Autodesk Fusion 360 part; units mm, degrees
(part 6 of 9)
  spline S17 degree 5 poles (27.8077, 5.2259) (27.7982, 5.2278) (27.7791, 5.232) (27.7507, 5.2389) (27.7131, 5.2496) (27.6667, 5.2648) (27.6206, 5.2814) (27.5747, 5.2988) (27.529, 5.3167) (27.4833, 5.3349) (27.4376, 5.3534) (27.3921, 5.3724) (27.3468, 5.3919) (27.3016, 5.4121) (27.2567, 5.4329) (27.2119, 5.4544) (27.1672, 5.4764) (27.1227, 5.4988) (27.0784, 5.5216) (27.0341, 5.5447) (26.9899, 5.5683) (26.9459, 5.5922) (26.902, 5.6164) (26.8582, 5.6411) (26.8146, 5.6662) (26.771, 5.6917) (26.7277, 5.7176) (26.6844, 5.7438) (26.6412, 5.7703) (26.5982, 5.7972) (26.5553, 5.8244) (26.5125, 5.8519) (26.4698, 5.8797) (26.4272, 5.9079) (26.3848, 5.9363) (26.3425, 5.9651) (26.3003, 5.9942) (26.2582, 6.0236) (26.2162, 6.0533) (26.1743, 6.0833) (26.1326, 6.1136) (26.091, 6.1441) (26.0495, 6.1749) (26.0081, 6.2061) (25.9668, 6.2375) (25.9256, 6.2691) (25.8846, 6.3011) (25.8437, 6.3333) (25.8029, 6.3658) (25.7622, 6.3985) (25.7216, 6.4315) (25.6811, 6.4648) (25.6408, 6.4983) (25.6005, 6.5321) (25.5604, 6.5661) (25.5204, 6.6004) (25.4805, 6.6349) (25.4408, 6.6696) (25.4011, 6.7047) (25.3616, 6.7399) (25.3222, 6.7754) (25.2829, 6.8111) (25.2437, 6.8471) (25.2046, 6.8833) (25.1657, 6.9197) (25.1269, 6.9564) (25.0882, 6.9933) (25.0496, 7.0304) (25.0111, 7.0677) (24.9727, 7.1053) (24.9345, 7.1431) (24.904, 7.1735) (24.8812, 7.1964) (24.866, 7.2117) (24.8584, 7.2194) knots 0 0 0 0 0 0 0.01428571 0.02857143 0.04285714 0.05714286 0.07142857 0.08571429 0.1 0.11428571 0.12857143 0.14285714 0.15714286 0.17142857 0.18571429 0.2 0.21428571 0.22857143 0.24285714 0.25714286 0.27142857 0.28571429 0.3 0.31428571 0.32857143 0.34285714 0.35714286 0.37142857 0.38571429 0.4 0.41428571 0.42857143 0.44285714 0.45714286 0.47142857 0.48571429 0.5 0.51428571 0.52857143 0.54285714 0.55714286 0.57142857 0.58571429 0.6 0.61428571 0.62857143 0.64285714 0.65714286 0.67142857 0.68571429 0.7 0.71428571 0.72857143 0.74285714 0.75714286 0.77142857 0.78571429 0.8 0.81428571 0.82857143 0.84285714 0.85714286 0.87142857 0.88571429 0.9 0.91428571 0.92857143 0.94285714 0.95714286 0.97142857 0.98571429 1 1 1 1 1 1
  line L17 (27.8077, 5.2259) -> (27.9539, 5.196)
  arc A35 (28.7419, 4.0645) -> (27.9539, 5.196) centre (27.7535, 4.2163) ccw
  arc A36 (28.7419, 4.0645) -> (28.689, 3.6964) centre (48.0648, 1.0985) ccw
  arc A37 (27.6141, 2.8328) -> (28.689, 3.6964) centre (27.6978, 3.8293) ccw
  line L18 (27.6141, 2.8328) -> (27.4655, 2.8453)
  spline S18 degree 5 poles (27.4655, 2.8453) (27.4557, 2.8461) (27.4363, 2.8475) (27.407, 2.8489) (27.368, 2.8492) (27.3192, 2.8477) (27.2703, 2.8448) (27.2214, 2.841) (27.1724, 2.8367) (27.1234, 2.8321) (27.0744, 2.8272) (27.0254, 2.8218) (26.9764, 2.8159) (26.9274, 2.8092) (26.8784, 2.8019) (26.8294, 2.7939) (26.7803, 2.7854) (26.7313, 2.7764) (26.6823, 2.7671) (26.6333, 2.7573) (26.5843, 2.7472) (26.5353, 2.7367) (26.4864, 2.7257) (26.4374, 2.7144) (26.3885, 2.7026) (26.3395, 2.6904) (26.2906, 2.6778) (26.2417, 2.6649) (26.1928, 2.6516) (26.144, 2.6379) (26.0951, 2.6239) (26.0463, 2.6096) (25.9975, 2.5949) (25.9487, 2.5799) (25.9, 2.5645) (25.8513, 2.5488) (25.8026, 2.5328) (25.7539, 2.5165) (25.7053, 2.4998) (25.6567, 2.4828) (25.6081, 2.4655) (25.5595, 2.4479) (25.511, 2.43) (25.4625, 2.4118) (25.4141, 2.3933) (25.3657, 2.3746) (25.3173, 2.3555) (25.269, 2.3361) (25.2206, 2.3164) (25.1724, 2.2965) (25.1241, 2.2762) (25.0759, 2.2557) (25.0278, 2.2349) (24.9797, 2.2139) (24.9316, 2.1925) (24.8836, 2.1709) (24.8356, 2.149) (24.7876, 2.1269) (24.7397, 2.1045) (24.6919, 2.0818) (24.644, 2.0588) (24.5963, 2.0356) (24.5485, 2.0122) (24.5009, 1.9884) (24.4532, 1.9644) (24.4057, 1.9402) (24.3581, 1.9157) (24.3106, 1.891) (24.2632, 1.866) (24.2158, 1.8408) (24.1685, 1.8153) (24.1307, 1.7947) (24.1023, 1.7791) (24.0834, 1.7687) (24.074, 1.7635) knots 0 0 0 0 0 0 0.01428571 0.02857143 0.04285714 0.05714286 0.07142857 0.08571429 0.1 0.11428571 0.12857143 0.14285714 0.15714286 0.17142857 0.18571429 0.2 0.21428571 0.22857143 0.24285714 0.25714286 0.27142857 0.28571429 0.3 0.31428571 0.32857143 0.34285714 0.35714286 0.37142857 0.38571429 0.4 0.41428571 0.42857143 0.44285714 0.45714286 0.47142857 0.48571429 0.5 0.51428571 0.52857143 0.54285714 0.55714286 0.57142857 0.58571429 0.6 0.61428571 0.62857143 0.64285714 0.65714286 0.67142857 0.68571429 0.7 0.71428571 0.72857143 0.74285714 0.75714286 0.77142857 0.78571429 0.8 0.81428571 0.82857143 0.84285714 0.85714286 0.87142857 0.88571429 0.9 0.91428571 0.92857143 0.94285714 0.95714286 0.97142857 0.98571429 1 1 1 1 1 1
  arc A38 (24.074, 1.7635) -> (24.074, 0.4334) centre (48.0648, 1.0985) ccw
  spline S19 degree 5 poles (27.4655, -0.6484) (27.4557, -0.6492) (27.4363, -0.6506) (27.407, -0.6519) (27.368, -0.6523) (27.3192, -0.6508) (27.2703, -0.6479) (27.2214, -0.6441) (27.1724, -0.6398) (27.1234, -0.6352) (27.0744, -0.6303) (27.0254, -0.6249) (26.9764, -0.6189) (26.9274, -0.6123) (26.8784, -0.605) (26.8294, -0.597) (26.7803, -0.5885) (26.7313, -0.5795) (26.6823, -0.5701) (26.6333, -0.5604) (26.5843, -0.5503) (26.5353, -0.5398) (26.4864, -0.5288) (26.4374, -0.5175) (26.3885, -0.5057) (26.3395, -0.4935) (26.2906, -0.4809) (26.2417, -0.468) (26.1928, -0.4546) (26.144, -0.441) (26.0951, -0.427) (26.0463, -0.4127) (25.9975, -0.398) (25.9487, -0.383) (25.9, -0.3676) (25.8513, -0.3519) (25.8026, -0.3359) (25.7539, -0.3195) (25.7053, -0.3029) (25.6567, -0.2859) (25.6081, -0.2686) (25.5595, -0.251) (25.511, -0.2331) (25.4625, -0.2149) (25.4141, -0.1964) (25.3657, -0.1776) (25.3173, -0.1585) (25.269, -0.1392) (25.2206, -0.1195) (25.1724, -0.0995) (25.1241, -0.0793) (25.0759, -0.0588) (25.0278, -0.038) (24.9797, -0.0169) (24.9316, 0.0044) (24.8836, 0.026) (24.8356, 0.0479) (24.7876, 0.0701) (24.7397, 0.0925) (24.6919, 0.1152) (24.644, 0.1381) (24.5963, 0.1613) (24.5485, 0.1848) (24.5009, 0.2085) (24.4532, 0.2325) (24.4057, 0.2567) (24.3581, 0.2812) (24.3106, 0.306) (24.2632, 0.3309) (24.2158, 0.3562) (24.1685, 0.3817) (24.1307, 0.4023) (24.1023, 0.4178) (24.0834, 0.4282) (24.074, 0.4334) knots 0 0 0 0 0 0 0.01428571 0.02857143 0.04285714 0.05714286 0.07142857 0.08571429 0.1 0.11428571 0.12857143 0.14285714 0.15714286 0.17142857 0.18571429 0.2 0.21428571 0.22857143 0.24285714 0.25714286 0.27142857 0.28571429 0.3 0.31428571 0.32857143 0.34285714 0.35714286 0.37142857 0.38571429 0.4 0.41428571 0.42857143 0.44285714 0.45714286 0.47142857 0.48571429 0.5 0.51428571 0.52857143 0.54285714 0.55714286 0.57142857 0.58571429 0.6 0.61428571 0.62857143 0.64285714 0.65714286 0.67142857 0.68571429 0.7 0.71428571 0.72857143 0.74285714 0.75714286 0.77142857 0.78571429 0.8 0.81428571 0.82857143 0.84285714 0.85714286 0.87142857 0.88571429 0.9 0.91428571 0.92857143 0.94285714 0.95714286 0.97142857 0.98571429 1 1 1 1 1 1
  line L19 (27.4655, -0.6484) -> (27.6141, -0.6359)
  arc A39 (28.689, -1.4995) -> (27.6141, -0.6359) centre (27.6978, -1.6324) ccw
  arc A40 (28.689, -1.4995) -> (28.7419, -1.8676) centre (48.0648, 1.0985) ccw
  arc A41 (27.9539, -2.999) -> (28.7419, -1.8676) centre (27.7535, -2.0193) ccw
  line L20 (27.9539, -2.999) -> (27.8077, -3.0289)
  spline S20 degree 5 poles (27.8077, -3.0289) (27.7982, -3.0309) (27.7791, -3.035) (27.7507, -3.042) (27.7131, -3.0526) (27.6667, -3.0678) (27.6206, -3.0844) (27.5747, -3.1018) (27.529, -3.1197) (27.4833, -3.138) (27.4376, -3.1565) (27.3921, -3.1755) (27.3468, -3.195) (27.3016, -3.2152) (27.2567, -3.236) (27.2119, -3.2575) (27.1672, -3.2794) (27.1227, -3.3019) (27.0784, -3.3247) (27.0341, -3.3478) (26.9899, -3.3713) (26.9459, -3.3952) (26.902, -3.4195) (26.8582, -3.4442) (26.8146, -3.4693) (26.771, -3.4948) (26.7277, -3.5206) (26.6844, -3.5468) (26.6412, -3.5734) (26.5982, -3.6002) (26.5553, -3.6274) (26.5125, -3.6549) (26.4698, -3.6828) (26.4272, -3.7109) (26.3848, -3.7394) (26.3425, -3.7682) (26.3003, -3.7973) (26.2582, -3.8267) (26.2162, -3.8564) (26.1743, -3.8864) (26.1326, -3.9166) (26.091, -3.9472) (26.0495, -3.978) (26.0081, -4.0091) (25.9668, -4.0405) (25.9256, -4.0722) (25.8846, -4.1042) (25.8437, -4.1364) (25.8029, -4.1688) (25.7622, -4.2016) (25.7216, -4.2346) (25.6811, -4.2678) (25.6408, -4.3014) (25.6005, -4.3351) (25.5604, -4.3692) (25.5204, -4.4034) (25.4805, -4.438) (25.4408, -4.4727) (25.4011, -4.5077) (25.3616, -4.543) (25.3222, -4.5785) (25.2829, -4.6142) (25.2437, -4.6501) (25.2046, -4.6863) (25.1657, -4.7228) (25.1269, -4.7594) (25.0882, -4.7963) (25.0496, -4.8334) (25.0111, -4.8708) (24.9727, -4.9083) (24.9345, -4.9461) (24.904, -4.9765) (24.8812, -4.9994) (24.866, -5.0148) (24.8584, -5.0224) knots 0 0 0 0 0 0 0.01428571 0.02857143 0.04285714 0.05714286 0.07142857 0.08571429 0.1 0.11428571 0.12857143 0.14285714 0.15714286 0.17142857 0.18571429 0.2 0.21428571 0.22857143 0.24285714 0.25714286 0.27142857 0.28571429 0.3 0.31428571 0.32857143 0.34285714 0.35714286 0.37142857 0.38571429 0.4 0.41428571 0.42857143 0.44285714 0.45714286 0.47142857 0.48571429 0.5 0.51428571 0.52857143 0.54285714 0.55714286 0.57142857 0.58571429 0.6 0.61428571 0.62857143 0.64285714 0.65714286 0.67142857 0.68571429 0.7 0.71428571 0.72857143 0.74285714 0.75714286 0.77142857 0.78571429 0.8 0.81428571 0.82857143 0.84285714 0.85714286 0.87142857 0.88571429 0.9 0.91428571 0.92857143 0.94285714 0.95714286 0.97142857 0.98571429 1 1 1 1 1 1
  arc A42 (24.8584, -5.0224) -> (25.2332, -6.2986) centre (48.0648, 1.0985) ccw
  spline S21 degree 5 poles (28.792, -6.3811) (28.7829, -6.3847) (28.7646, -6.3915) (28.737, -6.401) (28.6996, -6.4123) (28.6523, -6.4246) (28.6046, -6.4356) (28.5566, -6.4458) (28.5084, -6.4555) (28.4601, -6.4648) (28.4117, -6.4739) (28.3632, -6.4825) (28.3145, -6.4906) (28.2656, -6.4981) (28.2165, -6.5048) (28.1672, -6.511) (28.1178, -6.5167) (28.0682, -6.5219) (28.0186, -6.5267) (27.9688, -6.5311) (27.9189, -6.5352) (27.869, -6.5389) (27.8189, -6.5422) (27.7687, -6.5451) (27.7184, -6.5476) (27.6681, -6.5497) (27.6176, -6.5514) (27.567, -6.5528) (27.5164, -6.5538) (27.4656, -6.5544) (27.4148, -6.5548) (27.364, -6.5548) (27.313, -6.5544) (27.262, -6.5538) (27.2109, -6.5527) (27.1597, -6.5514) (27.1085, -6.5498) (27.0572, -6.5478) (27.0058, -6.5455) (26.9544, -6.5429) (26.9029, -6.54) (26.8514, -6.5368) (26.7998, -6.5333) (26.7481, -6.5295) (26.6964, -6.5254) (26.6447, -6.521) (26.5929, -6.5163) (26.541, -6.5114) (26.4891, -6.5061) (26.4372, -6.5006) (26.3852, -6.4947) (26.3332, -6.4886) (26.2811, -6.4822) (26.229, -6.4756) (26.1769, -6.4687) (26.1247, -6.4614) (26.0725, -6.454) (26.0202, -6.4462) (25.968, -6.4382) (25.9157, -6.4299) (25.8633, -6.4214) (25.8109, -6.4126) (25.7585, -6.4035) (25.7061, -6.3942) (25.6536, -6.3846) (25.6012, -6.3747) (25.5487, -6.3646) (25.4961, -6.3543) (25.4436, -6.3436) (25.391, -6.3328) (25.3384, -6.3217) (25.2963, -6.3126) (25.2647, -6.3056) (25.2437, -6.301) (25.2332, -6.2986) knots 0 0 0 0 0 0 0.01428571 0.02857143 0.04285714 0.05714286 0.07142857 0.08571429 0.1 0.11428571 0.12857143 0.14285714 0.15714286 0.17142857 0.18571429 0.2 0.21428571 0.22857143 0.24285714 0.25714286 0.27142857 0.28571429 0.3 0.31428571 0.32857143 0.34285714 0.35714286 0.37142857 0.38571429 0.4 0.41428571 0.42857143 0.44285714 0.45714286 0.47142857 0.48571429 0.5 0.51428571 0.52857143 0.54285714 0.55714286 0.57142857 0.58571429 0.6 0.61428571 0.62857143 0.64285714 0.65714286 0.67142857 0.68571429 0.7 0.71428571 0.72857143 0.74285714 0.75714286 0.77142857 0.78571429 0.8 0.81428571 0.82857143 0.84285714 0.85714286 0.87142857 0.88571429 0.9 0.91428571 0.92857143 0.94285714 0.95714286 0.97142857 0.98571429 1 1 1 1 1 1
  line L21 (28.792, -6.3811) -> (28.9311, -6.3273)
  arc A43 (30.2058, -6.8531) -> (28.9311, -6.3273) centre (29.2922, -7.2598) ccw
  arc A44 (30.2058, -6.8531) -> (30.3603, -7.1913) centre (48.0648, 1.0985) ccw
  arc A45 (29.9229, -8.499) -> (30.3603, -7.1913) centre (29.4546, -7.6154) ccw
  line L22 (29.9229, -8.499) -> (29.7911, -8.5688)
  spline S22 degree 5 poles (29.7911, -8.5688) (29.7825, -8.5734) (29.7654, -8.5827) (29.74, -8.5974) (29.707, -8.6182) (29.6668, -8.6459) (29.6272, -8.6748) (29.5881, -8.7044) (29.5492, -8.7345) (29.5105, -8.7648) (29.472, -8.7955) (29.4336, -8.8265) (29.3956, -8.858) (29.358, -8.8901) (29.3207, -8.9228) (29.2838, -8.956) (29.2471, -8.9896) (29.2108, -9.0237) (29.1746, -9.0581) (29.1386, -9.0927) (29.1029, -9.1277) (29.0674, -9.1631) (29.0321, -9.1987) (28.997, -9.2348) (28.9622, -9.2712) (28.9277, -9.3079) (28.8933, -9.3449) (28.8592, -9.3822) (28.8252, -9.4198) (28.7915, -9.4577) (28.758, -9.4959) (28.7247, -9.5344) (28.6916, -9.5731) (28.6587, -9.6121) (28.626, -9.6514) (28.5935, -9.6909) (28.5612, -9.7307) (28.5291, -9.7708) (28.4972, -9.8111) (28.4654, -9.8517) (28.4339, -9.8925) (28.4026, -9.9335) (28.3715, -9.9748) (28.3405, -10.0163) (28.3097, -10.0581) (28.2792, -10.1001) (28.2488, -10.1423) (28.2186, -10.1847) (28.1886, -10.2274) (28.1588, -10.2703) (28.1291, -10.3134) (28.0997, -10.3567) (28.0704, -10.4002) (28.0413, -10.4439) (28.0124, -10.4879) (27.9837, -10.532) (27.9551, -10.5764) (27.9268, -10.621) (27.8986, -10.6657) (27.8706, -10.7107) (27.8428, -10.7558) (27.8151, -10.8012) (27.7877, -10.8467) (27.7604, -10.8925) (27.7333, -10.9384) (27.7064, -10.9845) (27.6796, -11.0308) (27.6531, -11.0773) (27.6267, -11.124) (27.6004, -11.1708) (27.5744, -11.2178) (27.5537, -11.2556) (27.5383, -11.284) (27.528, -11.303) (27.5229, -11.3125) knots 0 0 0 0 0 0 0.01428571 0.02857143 0.04285714 0.05714286 0.07142857 0.08571429 0.1 0.11428571 0.12857143 0.14285714 0.15714286 0.17142857 0.18571429 0.2 0.21428571 0.22857143 0.24285714 0.25714286 0.27142857 0.28571429 0.3 0.31428571 0.32857143 0.34285714 0.35714286 0.37142857 0.38571429 0.4 0.41428571 0.42857143 0.44285714 0.45714286 0.47142857 0.48571429 0.5 0.51428571 0.52857143 0.54285714 0.55714286 0.57142857 0.58571429 0.6 0.61428571 0.62857143 0.64285714 0.65714286 0.67142857 0.68571429 0.7 0.71428571 0.72857143 0.74285714 0.75714286 0.77142857 0.78571429 0.8 0.81428571 0.82857143 0.84285714 0.85714286 0.87142857 0.88571429 0.9 0.91428571 0.92857143 0.94285714 0.95714286 0.97142857 0.98571429 1 1 1 1 1 1
  arc A46 (27.5229, -11.3125) -> (28.242, -12.4314) centre (48.0648, 1.0985) ccw
  spline S23 degree 5 poles (31.68, -11.5079) (31.6722, -11.5139) (31.6566, -11.5256) (31.6327, -11.5425) (31.6001, -11.5639) (31.5582, -11.589) (31.5155, -11.613) (31.4723, -11.6363) (31.4288, -11.6591) (31.3851, -11.6817) (31.3412, -11.7041) (31.2971, -11.726) (31.2526, -11.7475) (31.2078, -11.7684) (31.1626, -11.7888) (31.117, -11.8086) (31.0712, -11.8279) (31.0251, -11.8469) (30.9788, -11.8655) (30.9323, -11.8838) (30.8856, -11.9017) (30.8387, -11.9194) (30.7916, -11.9367) (30.7443, -11.9536) (30.6968, -11.9701) (30.649, -11.9863) (30.601, -12.0022) (30.5529, -12.0177) (30.5046, -12.033) (30.4561, -12.0479) (30.4075, -12.0625) (30.3586, -12.0769) (30.3097, -12.0909) (30.2605, -12.1046) (30.2112, -12.118) (30.1617, -12.1312) (30.1121, -12.144) (30.0623, -12.1566) (30.0124, -12.1689) (29.9623, -12.1809) (29.9121, -12.1926) (29.8618, -12.204) (29.8113, -12.2152) (29.7606, -12.2261) (29.7099, -12.2367) (29.659, -12.2471) (29.608, -12.2572) (29.5568, -12.267) (29.5056, -12.2766) (29.4542, -12.2859) (29.4026, -12.295) (29.351, -12.3038) (29.2993, -12.3123) (29.2474, -12.3206) (29.1954, -12.3287) (29.1433, -12.3364) (29.0911, -12.344) (29.0388, -12.3513) (28.9864, -12.3583) (28.9338, -12.3651) (28.8812, -12.3717) (28.8285, -12.378) (28.7756, -12.384) (28.7227, -12.3898) (28.6697, -12.3954) (28.6165, -12.4007) (28.5633, -12.4058) (28.51, -12.4107) (28.4566, -12.4153) (28.4031, -12.4197) (28.3495, -12.4239) (28.3065, -12.427) (28.2743, -12.4292) (28.2528, -12.4307) (28.242, -12.4314) knots 0 0 0 0 0 0 0.01428571 0.02857143 0.04285714 0.05714286 0.07142857 0.08571429 0.1 0.11428571 0.12857143 0.14285714 0.15714286 0.17142857 0.18571429 0.2 0.21428571 0.22857143 0.24285714 0.25714286 0.27142857 0.28571429 0.3 0.31428571 0.32857143 0.34285714 0.35714286 0.37142857 0.38571429 0.4 0.41428571 0.42857143 0.44285714 0.45714286 0.47142857 0.48571429 0.5 0.51428571 0.52857143 0.54285714 0.55714286 0.57142857 0.58571429 0.6 0.61428571 0.62857143 0.64285714 0.65714286 0.67142857 0.68571429 0.7 0.71428571 0.72857143 0.74285714 0.75714286 0.77142857 0.78571429 0.8 0.81428571 0.82857143 0.84285714 0.85714286 0.87142857 0.88571429 0.9 0.91428571 0.92857143 0.94285714 0.95714286 0.97142857 0.98571429 1 1 1 1 1 1
  line L23 (31.68, -11.5079) -> (31.7982, -11.4171)
  arc A47 (33.1694, -11.5624) -> (31.7982, -11.4171) centre (32.4074, -12.2101) ccw
  arc A48 (33.1694, -11.5624) -> (33.4129, -11.8435) centre (48.0648, 1.0985) ccw
  arc A49 (33.3617, -13.2214) -> (33.4129, -11.8435) centre (32.6634, -12.5055) ccw
  line L24 (33.3617, -13.2214) -> (33.2549, -13.3255)
  spline S24 degree 5 poles (33.2549, -13.3255) (33.2479, -13.3323) (33.2341, -13.3461) (33.214, -13.3673) (33.1881, -13.3966) (33.1573, -13.4345) (33.1275, -13.4734) (33.0983, -13.5128) (33.0695, -13.5526) (33.0409, -13.5926) (33.0125, -13.6329) (32.9845, -13.6735) (32.9569, -13.7144) (32.9298, -13.7558) (32.9033, -13.7976) (32.8772, -13.8399) (32.8515, -13.8825) (32.8262, -13.9254) (32.8012, -13.9686) (32.7765, -14.012) (32.752, -14.0557) (32.7279, -14.0996) (32.7041, -14.1438) (32.6806, -14.1882) (32.6575, -14.2329) (32.6346, -14.2779) (32.6121, -14.3231) (32.5899, -14.3685) (32.5679, -14.4142) (32.5463, -14.46) (32.5248, -14.5061) (32.5037, -14.5524) (32.4829, -14.5989) (32.4623, -14.6456) (32.442, -14.6925) (32.4219, -14.7396) (32.4021, -14.7869) (32.3826, -14.8344) (32.3634, -14.882) (32.3444, -14.9299) (32.3256, -14.9779) (32.3071, -15.0261) (32.2889, -15.0745) (32.2709, -15.1231) (32.2531, -15.1718) (32.2356, -15.2207) (32.2184, -15.2698) (32.2014, -15.319) (32.1846, -15.3684) (32.168, -15.4179) (32.1518, -15.4676) (32.1357, -15.5175) (32.1199, -15.5675) (32.1043, -15.6177) (32.0889, -15.668) (32.0738, -15.7184) (32.0589, -15.769) (32.0443, -15.8198) (32.0298, -15.8707) (32.0156, -15.9217) (32.0017, -15.9728) (31.9879, -16.0241) (31.9744, -16.0756) (31.9611, -16.1272) (31.948, -16.1789) (31.9352, -16.2307) (31.9226, -16.2826) (31.9102, -16.3347) (31.898, -16.3869) (31.8861, -16.4393) (31.8743, -16.4917) (31.8651, -16.5338) (31.8583, -16.5654) (31.8538, -16.5865) (31.8516, -16.5971) knots 0 0 0 0 0 0 0.01428571 0.02857143 0.04285714 0.05714286 0.07142857 0.08571429 0.1 0.11428571 0.12857143 0.14285714 0.15714286 0.17142857 0.18571429 0.2 0.21428571 0.22857143 0.24285714 0.25714286 0.27142857 0.28571429 0.3 0.31428571 0.32857143 0.34285714 0.35714286 0.37142857 0.38571429 0.4 0.41428571 0.42857143 0.44285714 0.45714286 0.47142857 0.48571429 0.5 0.51428571 0.52857143 0.54285714 0.55714286 0.57142857 0.58571429 0.6 0.61428571 0.62857143 0.64285714 0.65714286 0.67142857 0.68571429 0.7 0.71428571 0.72857143 0.74285714 0.75714286 0.77142857 0.78571429 0.8 0.81428571 0.82857143 0.84285714 0.85714286 0.87142857 0.88571429 0.9 0.91428571 0.92857143 0.94285714 0.95714286 0.97142857 0.98571429 1 1 1 1 1 1
  arc A50 (31.8516, -16.5971) -> (32.8568, -17.4681) centre (48.0648, 1.0985) ccw
  spline S25 degree 5 poles (35.8953, -15.6134) (35.8895, -15.6213) (35.8778, -15.6369) (35.8597, -15.6599) (35.8344, -15.6896) (35.8013, -15.7255) (35.7671, -15.7606) (35.7322, -15.7951) (35.6969, -15.8293) (35.6613, -15.8633) (35.6255, -15.8971) (35.5894, -15.9306) (35.5528, -15.9637) (35.5156, -15.9964) (35.478, -16.0286) (35.4399, -16.0605) (35.4013, -16.0919) (35.3625, -16.1231) (35.3233, -16.154) (35.2838, -16.1847) (35.2441, -16.2151) (35.2041, -16.2452) (35.1637, -16.2751) (35.1231, -16.3046) (35.0821, -16.3339) (35.0409, -16.3629) (34.9993, -16.3916) (34.9575, -16.4201) (34.9155, -16.4483) (34.8732, -16.4763) (34.8306, -16.5041) (34.7878, -16.5316) (34.7447, -16.5588) (34.7014, -16.5858) (34.6579, -16.6126) (34.6141, -16.6392) (34.5701, -16.6655) (34.5259, -16.6915) (34.4815, -16.7174) (34.4368, -16.743) (34.3919, -16.7684) (34.3469, -16.7936) (34.3016, -16.8185) (34.2561, -16.8432) (34.2103, -16.8677) (34.1644, -16.892) (34.1183, -16.9161) (34.072, -16.9399) (34.0255, -16.9636) (33.9788, -16.987) (33.932, -17.0102) (33.8849, -17.0332) (33.8376, -17.056) (33.7902, -17.0785) (33.7426, -17.1009) (33.6948, -17.123) (33.6468, -17.145) (33.5987, -17.1667) (33.5504, -17.1882) (33.5019, -17.2095) (33.4532, -17.2307) (33.4044, -17.2516) (33.3554, -17.2723) (33.3063, -17.2928) (33.257, -17.313) (33.2075, -17.3331) (33.1579, -17.353) (33.1081, -17.3727) (33.0581, -17.3922) (33.008, -17.4115) (32.9578, -17.4305) (32.9174, -17.4457) (32.8871, -17.4569) (32.8669, -17.4643) (32.8568, -17.4681) knots 0 0 0 0 0 0 0.01428571 0.02857143 0.04285714 0.05714286 0.07142857 0.08571429 0.1 0.11428571 0.12857143 0.14285714 0.15714286 0.17142857 0.18571429 0.2 0.21428571 0.22857143 0.24285714 0.25714286 0.27142857 0.28571429 0.3 0.31428571 0.32857143 0.34285714 0.35714286 0.37142857 0.38571429 0.4 0.41428571 0.42857143 0.44285714 0.45714286 0.47142857 0.48571429 0.5 0.51428571 0.52857143 0.54285714 0.55714286 0.57142857 0.58571429 0.6 0.61428571 0.62857143 0.64285714 0.65714286 0.67142857 0.68571429 0.7 0.71428571 0.72857143 0.74285714 0.75714286 0.77142857 0.78571429 0.8 0.81428571 0.82857143 0.84285714 0.85714286 0.87142857 0.88571429 0.9 0.91428571 0.92857143 0.94285714 0.95714286 0.97142857 0.98571429 1 1 1 1 1 1
  line L25 (35.8953, -15.6134) -> (35.9832, -15.4929)
  arc A51 (37.3397, -15.2461) -> (35.9832, -15.4929) centre (36.7911, -16.0822) ccw
  arc A52 (37.3397, -15.2461) -> (37.6526, -15.4472) centre (48.0648, 1.0985) ccw
  arc A53 (37.9916, -16.7837) -> (37.6526, -15.4472) centre (37.12, -16.2935) ccw
  line L26 (37.9916, -16.7837) -> (37.9185, -16.9136)
  spline S26 degree 5 poles (37.9185, -16.9136) (37.9137, -16.9222) (37.9044, -16.9393) (37.891, -16.9653) (37.8745, -17.0007) (37.8556, -17.0457) (37.8379, -17.0914) (37.821, -17.1375) (37.8046, -17.1838) (37.7884, -17.2303) (37.7726, -17.2769) (37.7571, -17.3237) (37.7422, -17.3708) (37.7278, -17.4181) (37.7142, -17.4657) (37.701, -17.5136) (37.6884, -17.5618) (37.6762, -17.6101) (37.6644, -17.6585) (37.6529, -17.7072) (37.6417, -17.7559) (37.631, -17.8049) (37.6206, -17.854) (37.6105, -17.9032) (37.6009, -17.9526) (37.5917, -18.0022) (37.5828, -18.0519) (37.5743, -18.1018) (37.5661, -18.1518) (37.5582, -18.2019) (37.5506, -18.2521) (37.5434, -18.3025) (37.5365, -18.353) (37.5299, -18.4036) (37.5236, -18.4543) (37.5177, -18.5051) (37.512, -18.5561) (37.5067, -18.6072) (37.5016, -18.6583) (37.4969, -18.7096) (37.4924, -18.761) (37.4882, -18.8124) (37.4844, -18.864) (37.4808, -18.9156) (37.4775, -18.9674) (37.4745, -19.0193) (37.4717, -19.0712) (37.4693, -19.1232) (37.4671, -19.1753) (37.4652, -19.2275) (37.4635, -19.2798) (37.4622, -19.3322) (37.4611, -19.3846) (37.4603, -19.4371) (37.4597, -19.4897) (37.4594, -19.5424) (37.4594, -19.5951) (37.4596, -19.648) (37.4601, -19.7009) (37.4609, -19.7538) (37.4619, -19.8068) (37.4631, -19.8599) (37.4647, -19.9131) (37.4664, -19.9663) (37.4685, -20.0196) (37.4707, -20.073) (37.4733, -20.1264) (37.4761, -20.1798) (37.4791, -20.2334) (37.4824, -20.287) (37.4859, -20.3406) (37.4889, -20.3836) (37.4913, -20.4158) (37.4929, -20.4373) (37.4937, -20.4481) knots 0 0 0 0 0 0 0.01428571 0.02857143 0.04285714 0.05714286 0.07142857 0.08571429 0.1 0.11428571 0.12857143 0.14285714 0.15714286 0.17142857 0.18571429 0.2 0.21428571 0.22857143 0.24285714 0.25714286 0.27142857 0.28571429 0.3 0.31428571 0.32857143 0.34285714 0.35714286 0.37142857 0.38571429 0.4 0.41428571 0.42857143 0.44285714 0.45714286 0.47142857 0.48571429 0.5 0.51428571 0.52857143 0.54285714 0.55714286 0.57142857 0.58571429 0.6 0.61428571 0.62857143 0.64285714 0.65714286 0.67142857 0.68571429 0.7 0.71428571 0.72857143 0.74285714 0.75714286 0.77142857 0.78571429 0.8 0.81428571 0.82857143 0.84285714 0.85714286 0.87142857 0.88571429 0.9 0.91428571 0.92857143 0.94285714 0.95714286 0.97142857 0.98571429 1 1 1 1 1 1
  arc A54 (37.4937, -20.4481) -> (38.7036, -21.0006) centre (48.0648, 1.0985) ccw
  spline S27 degree 5 poles (41.0965, -18.365) (41.0932, -18.3742) (41.0864, -18.3925) (41.0755, -18.4196) (41.0596, -18.4553) (41.0379, -18.4991) (41.015, -18.5423) (40.9912, -18.5853) (40.967, -18.628) (40.9424, -18.6707) (40.9176, -18.7132) (40.8923, -18.7555) (40.8666, -18.7976) (40.8401, -18.8394) (40.8131, -18.881) (40.7855, -18.9223) (40.7574, -18.9633) (40.7289, -19.0042) (40.7, -19.0449) (40.6708, -19.0854) (40.6412, -19.1258) (40.6113, -19.1659) (40.581, -19.206) (40.5503, -19.2458) (40.5193, -19.2854) (40.4879, -19.3248) (40.4561, -19.3641) (40.424, -19.4032) (40.3916, -19.4421) (40.3589, -19.4809) (40.3259, -19.5195) (40.2926, -19.558) (40.2589, -19.5963) (40.225, -19.6344) (40.1908, -19.6723) (40.1563, -19.7101) (40.1214, -19.7478) (40.0864, -19.7853) (40.051, -19.8226) (40.0154, -19.8597) (39.9795, -19.8968) (39.9433, -19.9336) (39.9069, -19.9703) (39.8702, -20.0068) (39.8332, -20.0432) (39.796, -20.0795) (39.7585, -20.1155) (39.7208, -20.1515) (39.6829, -20.1872) (39.6447, -20.2229) (39.6062, -20.2583) (39.5676, -20.2937) (39.5286, -20.3288) (39.4895, -20.3638) (39.4501, -20.3987) (39.4105, -20.4334) (39.3706, -20.468) (39.3306, -20.5024) (39.2903, -20.5367) (39.2498, -20.5708) (39.209, -20.6047) (39.1681, -20.6386) (39.1269, -20.6722) (39.0855, -20.7057) (39.0439, -20.7391) (39.0021, -20.7723) (38.9601, -20.8054) (38.9178, -20.8383) (38.8754, -20.8711) (38.8328, -20.9037) (38.7899, -20.9361) (38.7555, -20.962) (38.7296, -20.9813) (38.7122, -20.9942) (38.7036, -21.0006) knots 0 0 0 0 0 0 0.01428571 0.02857143 0.04285714 0.05714286 0.07142857 0.08571429 0.1 0.11428571 0.12857143 0.14285714 0.15714286 0.17142857 0.18571429 0.2 0.21428571 0.22857143 0.24285714 0.25714286 0.27142857 0.28571429 0.3 0.31428571 0.32857143 0.34285714 0.35714286 0.37142857 0.38571429 0.4 0.41428571 0.42857143 0.44285714 0.45714286 0.47142857 0.48571429 0.5 0.51428571 0.52857143 0.54285714 0.55714286 0.57142857 0.58571429 0.6 0.61428571 0.62857143 0.64285714 0.65714286 0.67142857 0.68571429 0.7 0.71428571 0.72857143 0.74285714 0.75714286 0.77142857 0.78571429 0.8 0.81428571 0.82857143 0.84285714 0.85714286 0.87142857 0.88571429 0.9 0.91428571 0.92857143 0.94285714 0.95714286 0.97142857 0.98571429 1 1 1 1 1 1
  line L27 (41.0965, -18.365) -> (41.1469, -18.2246)
  arc A55 (42.379, -17.6056) -> (41.1469, -18.2246) centre (42.0881, -18.5624) ccw
  arc A56 (42.379, -17.6056) -> (42.7358, -17.7104) centre (48.0648, 1.0985) ccw
  arc A57 (43.4376, -18.8972) -> (42.7358, -17.7104) centre (42.4632, -18.6725) ccw
  line L28 (43.4376, -18.8972) -> (43.4041, -19.0426)
  spline S28 degree 5 poles (43.4041, -19.0426) (43.4019, -19.0521) (43.3978, -19.0712) (43.3923, -19.0999) (43.3864, -19.1385) (43.3809, -19.187) (43.3769, -19.2358) (43.3736, -19.2848) (43.3709, -19.3339) (43.3685, -19.383) (43.3664, -19.4322) (43.3648, -19.4815) (43.3637, -19.5308) (43.3633, -19.5803) (43.3636, -19.6299) (43.3645, -19.6795) (43.3659, -19.7292) (43.3678, -19.779) (43.3701, -19.8289) (43.3728, -19.8788) (43.3758, -19.9287) (43.3793, -19.9787) (43.3831, -20.0287) (43.3874, -20.0788) (43.3921, -20.1289) (43.3972, -20.1791) (43.4027, -20.2293) (43.4086, -20.2796) (43.4148, -20.3298) (43.4213, -20.3801) (43.4282, -20.4305) (43.4355, -20.4808) (43.4431, -20.5312) (43.451, -20.5816) (43.4593, -20.6321) (43.4679, -20.6825) (43.4768, -20.733) (43.4861, -20.7835) (43.4956, -20.834) (43.5055, -20.8845) (43.5157, -20.9351) (43.5262, -20.9856) (43.537, -21.0362) (43.5481, -21.0868) (43.5595, -21.1374) (43.5713, -21.188) (43.5833, -21.2386) (43.5956, -21.2892) (43.6082, -21.3398) (43.621, -21.3904) (43.6342, -21.4411) (43.6476, -21.4917) (43.6614, -21.5423) (43.6754, -21.5929) (43.6897, -21.6436) (43.7042, -21.6942) (43.719, -21.7448) (43.7342, -21.7954) (43.7495, -21.846) (43.7652, -21.8966) (43.7811, -21.9472) (43.7972, -21.9978) (43.8137, -22.0484) (43.8304, -22.0989) (43.8473, -22.1495) (43.8646, -22.2001) (43.882, -22.2506) (43.8998, -22.3011) (43.9178, -22.3516) (43.936, -22.4021) (43.9545, -22.4526) (43.9695, -22.493) (43.9808, -22.5232) (43.9885, -22.5434) (43.9923, -22.5535) knots 0 0 0 0 0 0 0.01428571 0.02857143 0.04285714 0.05714286 0.07142857 0.08571429 0.1 0.11428571 0.12857143 0.14285714 0.15714286 0.17142857 0.18571429 0.2 0.21428571 0.22857143 0.24285714 0.25714286 0.27142857 0.28571429 0.3 0.31428571 0.32857143 0.34285714 0.35714286 0.37142857 0.38571429 0.4 0.41428571 0.42857143 0.44285714 0.45714286 0.47142857 0.48571429 0.5 0.51428571 0.52857143 0.54285714 0.55714286 0.57142857 0.58571429 0.6 0.61428571 0.62857143 0.64285714 0.65714286 0.67142857 0.68571429 0.7 0.71428571 0.72857143 0.74285714 0.75714286 0.77142857 0.78571429 0.8 0.81428571 0.82857143 0.84285714 0.85714286 0.87142857 0.88571429 0.9 0.91428571 0.92857143 0.94285714 0.95714286 0.97142857 0.98571429 1 1 1 1 1 1
  arc A58 (43.9923, -22.5535) -> (45.3088, -22.7428) centre (48.0648, 1.0985) ccw
  spline S29 degree 5 poles (46.8623, -19.5398) (46.8617, -19.5495) (46.8603, -19.569) (46.8575, -19.5981) (46.8523, -19.6368) (46.8438, -19.6849) (46.834, -19.7329) (46.8233, -19.7808) (46.8121, -19.8286) (46.8005, -19.8765) (46.7887, -19.9243) (46.7764, -19.972) (46.7635, -20.0197) (46.75, -20.0672) (46.7357, -20.1147) (46.7209, -20.1621) (46.7055, -20.2094) (46.6896, -20.2566) (46.6734, -20.3038) (46.6567, -20.3509) (46.6397, -20.398) (46.6224, -20.445) (46.6046, -20.4919) (46.5864, -20.5387) (46.5677, -20.5855) (46.5487, -20.6322) (46.5293, -20.6788) (46.5095, -20.7254) (46.4894, -20.7719) (46.4689, -20.8183) (46.4481, -20.8647) (46.427, -20.9109) (46.4055, -20.9572) (46.3837, -21.0033) (46.3615, -21.0493) (46.3391, -21.0953) (46.3163, -21.1413) (46.2932, -21.1871) (46.2698, -21.2329) (46.246, -21.2786) (46.222, -21.3242) (46.1977, -21.3697) (46.1731, -21.4152) (46.1482, -21.4606) (46.123, -21.5059) (46.0975, -21.5512) (46.0717, -21.5964) (46.0456, -21.6415) (46.0193, -21.6865) (45.9927, -21.7314) (45.9658, -21.7763) (45.9386, -21.8211) (45.9112, -21.8658) (45.8835, -21.9104) (45.8555, -21.955) (45.8273, -21.9994) (45.7988, -22.0438) (45.77, -22.0881) (45.741, -22.1324) (45.7118, -22.1765) (45.6822, -22.2206) (45.6525, -22.2645) (45.6225, -22.3084) (45.5922, -22.3523) (45.5617, -22.396) (45.5309, -22.4396) (45.4999, -22.4832) (45.4687, -22.5267) (45.4372, -22.5701) (45.4054, -22.6134) (45.3735, -22.6566) (45.3477, -22.6911) (45.3283, -22.717) (45.3153, -22.7342) (45.3088, -22.7428) knots 0 0 0 0 0 0 0.01428571 0.02857143 0.04285714 0.05714286 0.07142857 0.08571429 0.1 0.11428571 0.12857143 0.14285714 0.15714286 0.17142857 0.18571429 0.2 0.21428571 0.22857143 0.24285714 0.25714286 0.27142857 0.28571429 0.3 0.31428571 0.32857143 0.34285714 0.35714286 0.37142857 0.38571429 0.4 0.41428571 0.42857143 0.44285714 0.45714286 0.47142857 0.48571429 0.5 0.51428571 0.52857143 0.54285714 0.55714286 0.57142857 0.58571429 0.6 0.61428571 0.62857143 0.64285714 0.65714286 0.67142857 0.68571429 0.7 0.71428571 0.72857143 0.74285714 0.75714286 0.77142857 0.78571429 0.8 0.81428571 0.82857143 0.84285714 0.85714286 0.87142857 0.88571429 0.9 0.91428571 0.92857143 0.94285714 0.95714286 0.97142857 0.98571429 1 1 1 1 1 1
  line L29 (46.8623, -19.5398) -> (46.8711, -19.3909)
  arc A59 (47.8788, -18.4499) -> (46.8711, -19.3909) centre (47.8693, -19.4498) ccw
  arc A60 (47.8788, -18.4499) -> (48.2507, -18.4499) centre (48.0648, 1.0985) ccw
  arc A61 (49.2585, -19.3909) -> (48.2507, -18.4499) centre (48.2602, -19.4498) ccw
  line L30 (49.2585, -19.3909) -> (49.2673, -19.5398)
  spline S30 degree 5 poles (49.2673, -19.5398) (49.2679, -19.5495) (49.2693, -19.569) (49.2721, -19.5981) (49.2773, -19.6368) (49.2857, -19.6849) (49.2956, -19.7329) (49.3063, -19.7808) (49.3175, -19.8286) (49.329, -19.8765) (49.3409, -19.9243) (49.3532, -19.972) (49.3661, -20.0197) (49.3796, -20.0672) (49.3938, -20.1147) (49.4087, -20.1621) (49.4241, -20.2094) (49.44, -20.2566) (49.4562, -20.3038) (49.4728, -20.3509) (49.4898, -20.398) (49.5072, -20.445) (49.525, -20.4919) (49.5432, -20.5387) (49.5618, -20.5855) (49.5809, -20.6322) (49.6003, -20.6788) (49.6201, -20.7254) (49.6402, -20.7719) (49.6606, -20.8183) (49.6814, -20.8647) (49.7026, -20.9109) (49.7241, -20.9572) (49.7459, -21.0033) (49.768, -21.0493) (49.7905, -21.0953) (49.8133, -21.1413) (49.8364, -21.1871) (49.8598, -21.2329) (49.8835, -21.2786) (49.9075, -21.3242) (49.9319, -21.3697) (49.9565, -21.4152) (49.9814, -21.4606) (50.0066, -21.5059) (50.0321, -21.5512) (50.0579, -21.5964) (50.0839, -21.6415) (50.1103, -21.6865) (50.1369, -21.7314) (50.1638, -21.7763) (50.1909, -21.8211) (50.2184, -21.8658) (50.2461, -21.9104) (50.274, -21.955) (50.3023, -21.9994) (50.3308, -22.0438) (50.3595, -22.0881) (50.3885, -22.1324) (50.4178, -22.1765) (50.4473, -22.2206) (50.4771, -22.2645) (50.5071, -22.3084) (50.5374, -22.3523) (50.5679, -22.396) (50.5987, -22.4396) (50.6297, -22.4832) (50.6609, -22.5267) (50.6924, -22.5701) (50.7241, -22.6134) (50.7561, -22.6566) (50.7818, -22.6911) (50.8013, -22.717) (50.8143, -22.7342) (50.8208, -22.7428) knots 0 0 0 0 0 0 0.01428571 0.02857143 0.04285714 0.05714286 0.07142857 0.08571429 0.1 0.11428571 0.12857143 0.14285714 0.15714286 0.17142857 0.18571429 0.2 0.21428571 0.22857143 0.24285714 0.25714286 0.27142857 0.28571429 0.3 0.31428571 0.32857143 0.34285714 0.35714286 0.37142857 0.38571429 0.4 0.41428571 0.42857143 0.44285714 0.45714286 0.47142857 0.48571429 0.5 0.51428571 0.52857143 0.54285714 0.55714286 0.57142857 0.58571429 0.6 0.61428571 0.62857143 0.64285714 0.65714286 0.67142857 0.68571429 0.7 0.71428571 0.72857143 0.74285714 0.75714286 0.77142857 0.78571429 0.8 0.81428571 0.82857143 0.84285714 0.85714286 0.87142857 0.88571429 0.9 0.91428571 0.92857143 0.94285714 0.95714286 0.97142857 0.98571429 1 1 1 1 1 1
  arc A62 (50.8208, -22.7428) -> (52.1373, -22.5535) centre (48.0648, 1.0985) ccw
  spline S31 degree 5 poles (52.7254, -19.0426) (52.7276, -19.0521) (52.7318, -19.0712) (52.7373, -19.0999) (52.7432, -19.1385) (52.7486, -19.187) (52.7527, -19.2358) (52.7559, -19.2848) (52.7587, -19.3339) (52.7611, -19.383) (52.7632, -19.4322) (52.7648, -19.4815) (52.7659, -19.5308) (52.7663, -19.5803) (52.766, -19.6299) (52.7651, -19.6795) (52.7636, -19.7292) (52.7617, -19.779) (52.7594, -19.8289) (52.7568, -19.8788) (52.7537, -19.9287) (52.7503, -19.9787) (52.7464, -20.0287) (52.7422, -20.0788) (52.7375, -20.1289) (52.7323, -20.1791) (52.7269, -20.2293) (52.721, -20.2796) (52.7148, -20.3298) (52.7082, -20.3801) (52.7013, -20.4305) (52.6941, -20.4808) (52.6865, -20.5312) (52.6786, -20.5816) (52.6703, -20.6321) (52.6617, -20.6825) (52.6528, -20.733) (52.6435, -20.7835) (52.6339, -20.834) (52.624, -20.8845) (52.6138, -20.9351) (52.6033, -20.9856) (52.5925, -21.0362) (52.5814, -21.0868) (52.57, -21.1374) (52.5583, -21.188) (52.5463, -21.2386) (52.534, -21.2892) (52.5214, -21.3398) (52.5085, -21.3904) (52.4954, -21.4411) (52.4819, -21.4917) (52.4682, -21.5423) (52.4542, -21.5929) (52.4399, -21.6436) (52.4253, -21.6942) (52.4105, -21.7448) (52.3954, -21.7954) (52.38, -21.846) (52.3644, -21.8966) (52.3485, -21.9472) (52.3323, -21.9978) (52.3159, -22.0484) (52.2992, -22.0989) (52.2822, -22.1495) (52.265, -22.2001) (52.2475, -22.2506) (52.2298, -22.3011) (52.2118, -22.3516) (52.1936, -22.4021) (52.1751, -22.4526) (52.1601, -22.493) (52.1487, -22.5232) (52.1411, -22.5434) (52.1373, -22.5535) knots 0 0 0 0 0 0 0.01428571 0.02857143 0.04285714 0.05714286 0.07142857 0.08571429 0.1 0.11428571 0.12857143 0.14285714 0.15714286 0.17142857 0.18571429 0.2 0.21428571 0.22857143 0.24285714 0.25714286 0.27142857 0.28571429 0.3 0.31428571 0.32857143 0.34285714 0.35714286 0.37142857 0.38571429 0.4 0.41428571 0.42857143 0.44285714 0.45714286 0.47142857 0.48571429 0.5 0.51428571 0.52857143 0.54285714 0.55714286 0.57142857 0.58571429 0.6 0.61428571 0.62857143 0.64285714 0.65714286 0.67142857 0.68571429 0.7 0.71428571 0.72857143 0.74285714 0.75714286 0.77142857 0.78571429 0.8 0.81428571 0.82857143 0.84285714 0.85714286 0.87142857 0.88571429 0.9 0.91428571 0.92857143 0.94285714 0.95714286 0.97142857 0.98571429 1 1 1 1 1 1
  line L31 (52.7254, -19.0426) -> (52.6919, -18.8972)
  arc A63 (53.3938, -17.7104) -> (52.6919, -18.8972) centre (53.6664, -18.6725) ccw
  arc A64 (53.3938, -17.7104) -> (53.7506, -17.6056) centre (48.0648, 1.0985) ccw
  arc A65 (54.9827, -18.2246) -> (53.7506, -17.6056) centre (54.0414, -18.5624) ccw
  line L32 (54.9827, -18.2246) -> (55.033, -18.365)
  spline S32 degree 5 poles (55.033, -18.365) (55.0363, -18.3742) (55.0432, -18.3925) (55.0541, -18.4196) (55.07, -18.4553) (55.0916, -18.4991) (55.1146, -18.5423) (55.1384, -18.5853) (55.1626, -18.628) (55.1871, -18.6707) (55.212, -18.7132) (55.2372, -18.7555) (55.263, -18.7976) (55.2894, -18.8394) (55.3164, -18.881) (55.344, -18.9223) (55.3722, -18.9633) (55.4007, -19.0042) (55.4296, -19.0449) (55.4588, -19.0854) (55.4883, -19.1258) (55.5183, -19.1659) (55.5485, -19.206) (55.5792, -19.2458) (55.6103, -19.2854) (55.6417, -19.3248) (55.6735, -19.3641) (55.7055, -19.4032) (55.738, -19.4421) (55.7707, -19.4809) (55.8037, -19.5195) (55.837, -19.558) (55.8706, -19.5963) (55.9046, -19.6344) (55.9388, -19.6723) (55.9733, -19.7101) (56.0081, -19.7478) (56.0432, -19.7853) (56.0786, -19.8226) (56.1142, -19.8597) (56.1501, -19.8968) (56.1863, -19.9336) (56.2227, -19.9703) (56.2594, -20.0068) (56.2963, -20.0432) (56.3336, -20.0795) (56.371, -20.1155) (56.4087, -20.1515) (56.4467, -20.1872) (56.4849, -20.2229) (56.5233, -20.2583) (56.562, -20.2937) (56.6009, -20.3288) (56.6401, -20.3638) (56.6795, -20.3987) (56.7191, -20.4334) (56.7589, -20.468) (56.799, -20.5024) (56.8393, -20.5367) (56.8798, -20.5708) (56.9205, -20.6047) (56.9615, -20.6386) (57.0027, -20.6722) (57.044, -20.7057) (57.0856, -20.7391) (57.1275, -20.7723) (57.1695, -20.8054) (57.2117, -20.8383) (57.2541, -20.8711) (57.2968, -20.9037) (57.3396, -20.9361) (57.3741, -20.962) (57.4, -20.9813) (57.4173, -20.9942) (57.426, -21.0006) knots 0 0 0 0 0 0 0.01428571 0.02857143 0.04285714 0.05714286 0.07142857 0.08571429 0.1 0.11428571 0.12857143 0.14285714 0.15714286 0.17142857 0.18571429 0.2 0.21428571 0.22857143 0.24285714 0.25714286 0.27142857 0.28571429 0.3 0.31428571 0.32857143 0.34285714 0.35714286 0.37142857 0.38571429 0.4 0.41428571 0.42857143 0.44285714 0.45714286 0.47142857 0.48571429 0.5 0.51428571 0.52857143 0.54285714 0.55714286 0.57142857 0.58571429 0.6 0.61428571 0.62857143 0.64285714 0.65714286 0.67142857 0.68571429 0.7 0.71428571 0.72857143 0.74285714 0.75714286 0.77142857 0.78571429 0.8 0.81428571 0.82857143 0.84285714 0.85714286 0.87142857 0.88571429 0.9 0.91428571 0.92857143 0.94285714 0.95714286 0.97142857 0.98571429 1 1 1 1 1 1
  arc A66 (57.426, -21.0006) -> (58.6358, -20.4481) centre (48.0648, 1.0985) ccw
  spline S33 degree 5 poles (58.211, -16.9136) (58.2158, -16.9222) (58.2252, -16.9393) (58.2385, -16.9653) (58.2551, -17.0007) (58.274, -17.0457) (58.2917, -17.0914) (58.3085, -17.1375) (58.325, -17.1838) (58.3411, -17.2303) (58.357, -17.2769) (58.3725, -17.3237) (58.3874, -17.3708) (58.4017, -17.4181) (58.4154, -17.4657) (58.4285, -17.5136) (58.4412, -17.5618) (58.4533, -17.6101) (58.4652, -17.6585) (58.4767, -17.7072) (58.4878, -17.7559) (58.4986, -17.8049) (58.509, -17.854) (58.519, -17.9032) (58.5286, -17.9526) (58.5379, -18.0022) (58.5467, -18.0519) (58.5553, -18.1018) (58.5635, -18.1518) (58.5714, -18.2019) (58.5789, -18.2521) (58.5862, -18.3025) (58.5931, -18.353) (58.5997, -18.4036) (58.6059, -18.4543) (58.6119, -18.5051) (58.6175, -18.5561) (58.6229, -18.6072) (58.6279, -18.6583) (58.6327, -18.7096) (58.6371, -18.761) (58.6413, -18.8124) (58.6452, -18.864) (58.6488, -18.9156) (58.6521, -18.9674) (58.6551, -19.0193) (58.6578, -19.0712) (58.6603, -19.1232) (58.6625, -19.1753) (58.6644, -19.2275) (58.666, -19.2798) (58.6674, -19.3322) (58.6685, -19.3846) (58.6693, -19.4371) (58.6698, -19.4897) (58.6701, -19.5424) (58.6702, -19.5951) (58.6699, -19.648) (58.6694, -19.7009) (58.6687, -19.7538) (58.6677, -19.8068) (58.6664, -19.8599) (58.6649, -19.9131) (58.6631, -19.9663) (58.6611, -20.0196) (58.6588, -20.073) (58.6563, -20.1264) (58.6535, -20.1798) (58.6505, -20.2334) (58.6472, -20.287) (58.6437, -20.3406) (58.6407, -20.3836) (58.6383, -20.4158) (58.6367, -20.4373) (58.6358, -20.4481) knots 0 0 0 0 0 0 0.01428571 0.02857143 0.04285714 0.05714286 0.07142857 0.08571429 0.1 0.11428571 0.12857143 0.14285714 0.15714286 0.17142857 0.18571429 0.2 0.21428571 0.22857143 0.24285714 0.25714286 0.27142857 0.28571429 0.3 0.31428571 0.32857143 0.34285714 0.35714286 0.37142857 0.38571429 0.4 0.41428571 0.42857143 0.44285714 0.45714286 0.47142857 0.48571429 0.5 0.51428571 0.52857143 0.54285714 0.55714286 0.57142857 0.58571429 0.6 0.61428571 0.62857143 0.64285714 0.65714286 0.67142857 0.68571429 0.7 0.71428571 0.72857143 0.74285714 0.75714286 0.77142857 0.78571429 0.8 0.81428571 0.82857143 0.84285714 0.85714286 0.87142857 0.88571429 0.9 0.91428571 0.92857143 0.94285714 0.95714286 0.97142857 0.98571429 1 1 1 1 1 1
  line L33 (58.211, -16.9136) -> (58.1379, -16.7837)
  arc A67 (58.477, -15.4472) -> (58.1379, -16.7837) centre (59.0096, -16.2935) ccw
  arc A68 (58.477, -15.4472) -> (58.7898, -15.2461) centre (48.0648, 1.0985) ccw
  arc A69 (60.1464, -15.4929) -> (58.7898, -15.2461) centre (59.3384, -16.0822) ccw
  line L34 (60.1464, -15.4929) -> (60.2343, -15.6134)
  spline S34 degree 5 poles (60.2343, -15.6134) (60.24, -15.6213) (60.2517, -15.6369) (60.2699, -15.6599) (60.2951, -15.6896) (60.3283, -15.7255) (60.3625, -15.7606) (60.3974, -15.7951) (60.4327, -15.8293) (60.4682, -15.8633) (60.504, -15.8971) (60.5402, -15.9306) (60.5768, -15.9637) (60.6139, -15.9964) (60.6516, -16.0286) (60.6897, -16.0605) (60.7282, -16.0919) (60.7671, -16.1231) (60.8063, -16.154) (60.8457, -16.1847) (60.8855, -16.2151) (60.9255, -16.2452) (60.9658, -16.2751) (61.0065, -16.3046) (61.0474, -16.3339) (61.0887, -16.3629) (61.1302, -16.3916) (61.172, -16.4201) (61.2141, -16.4483) (61.2564, -16.4763) (61.299, -16.5041) (61.3418, -16.5316) (61.3848, -16.5588) (61.4281, -16.5858) (61.4716, -16.6126) (61.5154, -16.6392) (61.5594, -16.6655) (61.6036, -16.6915) (61.6481, -16.7174) (61.6927, -16.743) (61.7376, -16.7684) (61.7827, -16.7936) (61.828, -16.8185) (61.8735, -16.8432) (61.9192, -16.8677) (61.9651, -16.892) (62.0112, -16.9161) (62.0575, -16.9399) (62.104, -16.9636) (62.1507, -16.987) (62.1976, -17.0102) (62.2447, -17.0332) (62.2919, -17.056) (62.3393, -17.0785) (62.387, -17.1009) (62.4347, -17.123) (62.4827, -17.145) (62.5309, -17.1667) (62.5792, -17.1882) (62.6277, -17.2095) (62.6763, -17.2307) (62.7251, -17.2516) (62.7741, -17.2723) (62.8233, -17.2928) (62.8726, -17.313) (62.9221, -17.3331) (62.9717, -17.353) (63.0215, -17.3727) (63.0714, -17.3922) (63.1215, -17.4115) (63.1718, -17.4305) (63.2121, -17.4457) (63.2424, -17.4569) (63.2627, -17.4643) (63.2728, -17.4681) knots 0 0 0 0 0 0 0.01428571 0.02857143 0.04285714 0.05714286 0.07142857 0.08571429 0.1 0.11428571 0.12857143 0.14285714 0.15714286 0.17142857 0.18571429 0.2 0.21428571 0.22857143 0.24285714 0.25714286 0.27142857 0.28571429 0.3 0.31428571 0.32857143 0.34285714 0.35714286 0.37142857 0.38571429 0.4 0.41428571 0.42857143 0.44285714 0.45714286 0.47142857 0.48571429 0.5 0.51428571 0.52857143 0.54285714 0.55714286 0.57142857 0.58571429 0.6 0.61428571 0.62857143 0.64285714 0.65714286 0.67142857 0.68571429 0.7 0.71428571 0.72857143 0.74285714 0.75714286 0.77142857 0.78571429 0.8 0.81428571 0.82857143 0.84285714 0.85714286 0.87142857 0.88571429 0.9 0.91428571 0.92857143 0.94285714 0.95714286 0.97142857 0.98571429 1 1 1 1 1 1
  arc A70 (63.2728, -17.4681) -> (64.278, -16.5971) centre (48.0648, 1.0985) ccw
  spline S35 degree 5 poles (62.8746, -13.3255) (62.8816, -13.3323) (62.8954, -13.3461) (62.9156, -13.3673) (62.9414, -13.3966) (62.9723, -13.4345) (63.0021, -13.4734) (63.0312, -13.5128) (63.0601, -13.5526) (63.0887, -13.5926) (63.117, -13.6329) (63.145, -13.6735) (63.1726, -13.7144) (63.1997, -13.7558) (63.2263, -13.7976) (63.2524, -13.8399) (63.278, -13.8825) (63.3033, -13.9254) (63.3284, -13.9686) (63.3531, -14.012) (63.3775, -14.0557) (63.4016, -14.0996) (63.4255, -14.1438) (63.4489, -14.1882) (63.4721, -14.2329) (63.4949, -14.2779) (63.5174, -14.3231) (63.5397, -14.3685) (63.5616, -14.4142) (63.5833, -14.46) (63.6047, -14.5061) (63.6258, -14.5524) (63.6467, -14.5989) (63.6673, -14.6456) (63.6876, -14.6925) (63.7076, -14.7396) (63.7274, -14.7869) (63.7469, -14.8344) (63.7662, -14.882) (63.7852, -14.9299) (63.8039, -14.9779) (63.8224, -15.0261) (63.8407, -15.0745) (63.8587, -15.1231) (63.8764, -15.1718) (63.8939, -15.2207) (63.9112, -15.2698) (63.9282, -15.319) (63.945, -15.3684) (63.9615, -15.4179) (63.9778, -15.4676) (63.9939, -15.5175) (64.0097, -15.5675) (64.0253, -15.6177) (64.0406, -15.668) (64.0558, -15.7184) (64.0706, -15.769) (64.0853, -15.8198) (64.0997, -15.8707) (64.1139, -15.9217) (64.1279, -15.9728) (64.1416, -16.0241) (64.1552, -16.0756) (64.1684, -16.1272) (64.1815, -16.1789) (64.1944, -16.2307) (64.207, -16.2826) (64.2194, -16.3347) (64.2316, -16.3869) (64.2435, -16.4393) (64.2552, -16.4917) (64.2645, -16.5338) (64.2713, -16.5654) (64.2758, -16.5865) (64.278, -16.5971) knots 0 0 0 0 0 0 0.01428571 0.02857143 0.04285714 0.05714286 0.07142857 0.08571429 0.1 0.11428571 0.12857143 0.14285714 0.15714286 0.17142857 0.18571429 0.2 0.21428571 0.22857143 0.24285714 0.25714286 0.27142857 0.28571429 0.3 0.31428571 0.32857143 0.34285714 0.35714286 0.37142857 0.38571429 0.4 0.41428571 0.42857143 0.44285714 0.45714286 0.47142857 0.48571429 0.5 0.51428571 0.52857143 0.54285714 0.55714286 0.57142857 0.58571429 0.6 0.61428571 0.62857143 0.64285714 0.65714286 0.67142857 0.68571429 0.7 0.71428571 0.72857143 0.74285714 0.75714286 0.77142857 0.78571429 0.8 0.81428571 0.82857143 0.84285714 0.85714286 0.87142857 0.88571429 0.9 0.91428571 0.92857143 0.94285714 0.95714286 0.97142857 0.98571429 1 1 1 1 1 1
  line L35 (62.8746, -13.3255) -> (62.7679, -13.2214)
  arc A71 (62.7166, -11.8435) -> (62.7679, -13.2214) centre (63.4661, -12.5055) ccw
  arc A72 (62.7166, -11.8435) -> (62.9602, -11.5624) centre (48.0648, 1.0985) ccw
  arc A73 (64.3313, -11.4171) -> (62.9602, -11.5624) centre (63.7221, -12.2101) ccw
  line L36 (64.3313, -11.4171) -> (64.4496, -11.5079)
  spline S36 degree 5 poles (64.4496, -11.5079) (64.4573, -11.5139) (64.473, -11.5256) (64.4968, -11.5425) (64.5295, -11.5639) (64.5714, -11.589) (64.6141, -11.613) (64.6573, -11.6363) (64.7008, -11.6591) (64.7445, -11.6817) (64.7884, -11.7041) (64.8325, -11.726) (64.8769, -11.7475) (64.9218, -11.7684) (64.967, -11.7888) (65.0125, -11.8086) (65.0584, -11.8279) (65.1044, -11.8469) (65.1507, -11.8655) (65.1972, -11.8838) (65.2439, -11.9017) (65.2908, -11.9194) (65.3379, -11.9367) (65.3853, -11.9536) (65.4328, -11.9701) (65.4806, -11.9863) (65.5285, -12.0022) (65.5766, -12.0177) (65.625, -12.033) (65.6734, -12.0479) (65.7221, -12.0625) (65.7709, -12.0769) (65.8199, -12.0909) (65.8691, -12.1046) (65.9184, -12.118) (65.9678, -12.1312) (66.0175, -12.144) (66.0672, -12.1566) (66.1172, -12.1689) (66.1672, -12.1809) (66.2175, -12.1926) (66.2678, -12.204) (66.3183, -12.2152) (66.3689, -12.2261) (66.4197, -12.2367) (66.4706, -12.2471) (66.5216, -12.2572) (66.5727, -12.267) (66.624, -12.2766) (66.6754, -12.2859) (66.7269, -12.295) (66.7786, -12.3038) (66.8303, -12.3123) (66.8822, -12.3206) (66.9342, -12.3287) (66.9863, -12.3364) (67.0385, -12.344) (67.0908, -12.3513) (67.1432, -12.3583) (67.1957, -12.3651) (67.2484, -12.3717) (67.3011, -12.378) (67.3539, -12.384) (67.4069, -12.3898) (67.4599, -12.3954) (67.513, -12.4007) (67.5663, -12.4058) (67.6196, -12.4107) (67.673, -12.4153) (67.7265, -12.4197) (67.7801, -12.4239) (67.823, -12.427) (67.8553, -12.4292) (67.8768, -12.4307) (67.8876, -12.4314) knots 0 0 0 0 0 0 0.01428571 0.02857143 0.04285714 0.05714286 0.07142857 0.08571429 0.1 0.11428571 0.12857143 0.14285714 0.15714286 0.17142857 0.18571429 0.2 0.21428571 0.22857143 0.24285714 0.25714286 0.27142857 0.28571429 0.3 0.31428571 0.32857143 0.34285714 0.35714286 0.37142857 0.38571429 0.4 0.41428571 0.42857143 0.44285714 0.45714286 0.47142857 0.48571429 0.5 0.51428571 0.52857143 0.54285714 0.55714286 0.57142857 0.58571429 0.6 0.61428571 0.62857143 0.64285714 0.65714286 0.67142857 0.68571429 0.7 0.71428571 0.72857143 0.74285714 0.75714286 0.77142857 0.78571429 0.8 0.81428571 0.82857143 0.84285714 0.85714286 0.87142857 0.88571429 0.9 0.91428571 0.92857143 0.94285714 0.95714286 0.97142857 0.98571429 1 1 1 1 1 1
  arc A74 (67.8876, -12.4314) -> (68.6067, -11.3125) centre (48.0648, 1.0985) ccw